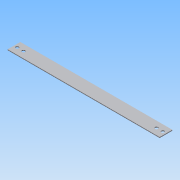
# Autodesk Inventor part: FrameMember
Saved by Autodesk Inventor 2014 (Build 180170000, 170)
## iProperties
Created: 2012-05-22
Part Number: FrameMember
Material: Aluminum 6061
Document SubType Name: Modeling
Designer: dgitz
Density: 1 g/cm^3
Appearance: Aluminum - Flat
d0: 1.000 in
d1: 12.000 in
d2: 0.063 in
d3: 0.00 deg
Author: dgitz
Autodesk Inventor part; units mm, degrees
ref_plane "YZ Plane" through (0, 0, 0) normal (1, 0, 0) x (0, 1, 0)
ref_plane "XZ Plane" through (0, 0, 0) normal (0, 1, 0) x (-1, 0, 0)
ref_plane "XY Plane" through (0, 0, 0) normal (0, 0, 1) x (1, 0, 0)
sketch "Sketch2" plane through (0, 0, 0) normal (0, 1, 0) x (-1, 0, 0)
  line L0 (-152.4, 12.7) -> (152.4, 12.7)
  line L1 (152.4, 12.7) -> (152.4, -12.7)
  line L2 (152.4, -12.7) -> (-152.4, -12.7)
  line L3 (-152.4, -12.7) -> (-152.4, 12.7)
  line L4 (-152.4, 12.7) -> (152.4, -12.7) construction
  point P0 (0, 0)
  point P1 (0, 0)
  dimension "d0" = 25.4
  dimension "d1" = 304.8
  constraints: 10 end point, 2 parallel, 1 coincident, 1 horizontal, 1 midpoint, 1 perpendicular
  measures "d0" distance between parallel lines of L2 L0
  measures "d1" distance of L0.start L0.end
extrude "Extrusion1" add sketch "Sketch2" along normal blind 1.5875
sketch "Sketch3" plane through (0, 0, 0) normal (0, -1, 0) x (1, 0, 0)
  line L0 (152.4, 12.7) -> (-152.4, 12.7) projected
  line L1 (-152.4, -12.7) -> (152.4, -12.7) projected
  line L2 (152.4, -12.7) -> (152.4, 12.7) projected
  line L3 (152.4, 0) -> (133.0754, 0) construction
  line L4 (0, 12.7) -> (0, -12.7) construction
  circle A0 centre (146.05, 0) radius 3.175
  circle A1 centre (133.35, 0) radius 3.175
  circle A2 centre (-146.05, 0) radius 3.175
  circle A3 centre (-133.35, 0) radius 3.175
  point P0 (0, 0)
  dimension "d4" = 6.35
  dimension "d5" = 6.35
  dimension "d6" = 12.7
  constraints: 4 centre point, 4 end point, 3 midpoint, 2 symmetric about line, 1 equal radius, 1 perpendicular, 1 point on line, 2 other
  measures "d4" diameter of A0
  measures "d5" distance from line of L2 A0.centre
  measures "d6" distance of A0.centre A1.centre
extrude "Extrusion2" cut sketch "Sketch3" against normal up to next
body "Solid1"
